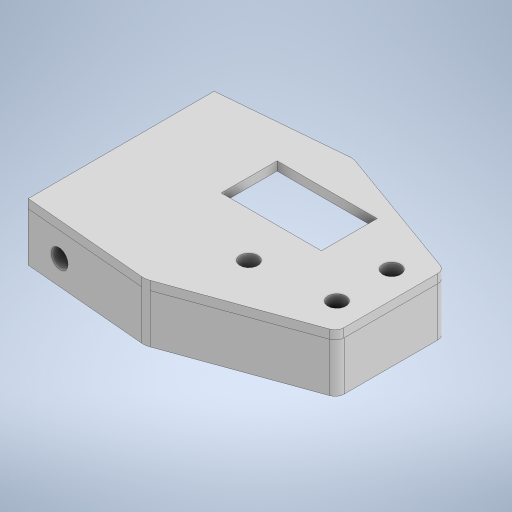
# Autodesk Inventor part: base_edited
Saved by Autodesk Inventor 2023 (Build 270158000, 158)
## iProperties
Created: 2024-05-12
Part Number: base_edited
Material: Ogólny
Document SubType Name: Modeling
Designer: kamil
Density: 1 g/cm^3
Appearance: Domyślna
Author: kamil
Autodesk Inventor part; units mm, degrees
ref_plane "YZ Plane" through (0, 0, 0) normal (1, 0, 0) x (0, 1, 0)
ref_plane "XZ Plane" through (0, 0, 0) normal (0, 1, 0) x (-1, 0, 0)
ref_plane "XY Plane" through (0, 0, 0) normal (0, 0, 1) x (1, 0, 0)
sketch "Szkic1" plane through (0, 0, 0) normal (0, 1, 0) x (-1, 0, 0)
  line L0 (0, 0) -> (0, 42)
  line L1 (-28.0748, -2.4593) -> (0, 0)
  line L2 (-59.6141, 8.5234) -> (-29.7811, -2.2373)
  circle A0 centre (-54.9356, 14.8089) radius 2.0248
  circle A1 centre (-54.9355, 27.1912) radius 2.0249
  circle A2 centre (-37.047, 29.1912) radius 2.025
  line L3 (0, 42) -> (-28.0748, 44.4593)
  line L4 (-29.7811, 44.2372) -> (-59.6141, 33.4766)
  circle A3 centre (-28.4239, 40.4745) radius 4.0001
  circle A4 centre (-58.9355, 31.5953) radius 2
  line L5 (-60.9355, 31.5953) -> (-60.9355, 10.4047)
  circle A5 centre (-58.9355, 10.4047) radius 2
  circle A6 centre (-28.4239, 1.5252) radius 3.9998
  line L6 (-43.3459, 19.1078) -> (-20.7459, 19.1078)
  line L7 (-20.7459, 19.1078) -> (-20.7459, 6.5098)
  line L8 (-20.7459, 6.5098) -> (-43.3459, 6.5098)
  line L9 (-43.3459, 6.5098) -> (-43.3459, 19.1078)
  point P0 (-40, 21)
  constraints: 20 end point, 7 centre point
extrude "Wyciągnięcie proste1" add sketch "Szkic1" along normal blind 2
sketch "Szkic2" plane through (0, 0, 0) normal (0, -1, 0) x (1, 0, 0)
  line L0 (4.5002, 37.877) -> (28.9526, 40.019)
  line L1 (28.9526, 19.1078) -> (28.9526, 40.019)
  line L2 (43.3459, 19.1078) -> (48.2961, 19.1078)
  line L3 (48.2961, 6.5098) -> (48.2961, 19.1078)
  line L4 (43.3461, 2.6556) -> (43.3461, 6.5098)
  line L5 (48.2961, 6.5098) -> (43.3459, 6.5098)
  circle A0 centre (58.9357, 10.4048) radius 2
  line L6 (59.6143, 33.4767) -> (59.5948, 33.4837)
  circle A1 centre (58.9355, 31.5953) radius 2.0002
  line L7 (4.5002, 37.877) -> (4.5002, -0.3941)
  line L8 (28.075, -2.4592) -> (28.052, -2.4572)
  arc A2 (60.9355, 31.5953) -> (59.6141, 33.4766) centre (58.9355, 31.5953) ccw projected
  arc A3 (59.6141, 8.5234) -> (60.9355, 10.4047) centre (58.9355, 10.4047) ccw projected
  circle A4 centre (37.047, 29.1912) radius 2.025 projected
  circle A5 centre (54.9356, 14.8089) radius 2.0248 projected
  circle A6 centre (54.9355, 27.1912) radius 2.0249 projected
  line L9 (0, 42) -> (28.0748, 44.4593) projected
  line L10 (0, 0) -> (0, 42) projected
  line L11 (28.0748, -2.4593) -> (0, 0) projected
  arc A7 (28.0748, -2.4593) -> (29.7811, -2.2372) centre (28.4239, 1.5252) ccw projected
  line L12 (59.6141, 8.5234) -> (29.7811, -2.2372) projected
  arc A8 (59.6141, 8.5234) -> (60.9355, 10.4047) centre (58.9355, 10.4047) ccw projected
  line L13 (60.9355, 31.5953) -> (60.9355, 10.4047) projected
  arc A9 (60.9355, 31.5953) -> (59.6141, 33.4766) centre (58.9355, 31.5953) ccw projected
  line L14 (29.7811, 44.2372) -> (59.6141, 33.4766) projected
  arc A10 (29.7811, 44.2372) -> (28.0748, 44.4593) centre (28.4239, 40.4745) ccw projected
  circle A11 centre (37.047, 29.1912) radius 2.025 projected
  circle A12 centre (54.9356, 14.8089) radius 2.0248 projected
  circle A13 centre (54.9355, 27.1912) radius 2.0249 projected
  line L15 (43.3459, 6.5098) -> (43.3459, 19.1078) projected
  line L16 (20.7459, 6.5098) -> (43.3459, 6.5098) projected
  line L17 (20.7459, 19.1078) -> (20.7459, 6.5098) projected
  line L18 (43.3459, 19.1078) -> (20.7459, 19.1078) projected
  line L19 (4.5002, -0.3941) -> (4.5002, -2.2372)
  line L20 (28.9526, 19.1078) -> (28.9526, 16.8338)
  line L21 (43.3459, 6.5098) -> (42.3677, 6.5098)
  line L22 (43.3459, 6.5098) -> (43.3459, 8.4048)
  line L23 (43.3459, 6.5098) -> (43.3459, 19.1078) projected
  line L24 (43.3459, 19.1078) -> (42.3677, 19.1078)
  line L25 (43.3459, 19.1078) -> (43.3459, 17.9708)
  point P0 (40.0002, 21.0001)
  point P1 (59.6047, 8.52)
  point P2 (60.9355, 10.4349)
  point P3 (60.9355, 31.5648)
  point P4 (59.5854, 33.487)
  point P5 (4.5002, -0.3942)
  point P6 (28.9526, 19.1078)
  point P7 (43.3461, 2.6556)
  constraints: 28 end point, 7 point on line, 1 centre point, 1 point on circle, 1 vertical, 6 other
extrude "Wyciągnięcie proste2" add sketch "Szkic2" along normal blind 11.024 contours L7 L11 L10 L9 A10 L14 A1 L13 A0 L12 L4 L5 L3 L2 L18 L1 L0 | A0 | L6 A1
sketch "Szkic3" plane through (43.3459, 2, 19.1078) normal (0, 0, -1) x (-1, 0, 0)
  circle A0 centre (35.5684, -7.5107) radius 2.1003
  point P0 (43.3459, -2)
  constraints: 1 centre point
extrude "Wyciągnięcie proste3" cut sketch "Szkic3" against normal through all
